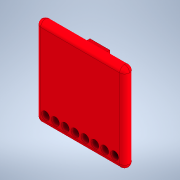
# Autodesk Inventor part: Czujnik GPS ZOE-M8Q
Saved by Autodesk Inventor 2020 (Build 240168000, 168)
## iProperties
Created: 2021-10-10
Part Number: Czujnik GPS ZOE-M8Q
Material: Ogólny
Document SubType Name: Modeling
Designer: Komputer
Density: 1 g/cm^3
Appearance: Domyślna
Author: Komputer
Autodesk Inventor part; units mm, degrees
ref_plane "YZ Plane" through (0, 0, 0) normal (1, 0, 0) x (0, 1, 0)
ref_plane "XZ Plane" through (0, 0, 0) normal (0, 1, 0) x (-1, 0, 0)
ref_plane "XY Plane" through (0, 0, 0) normal (0, 0, 1) x (1, 0, 0)
sketch "Szkic1" plane through (0, 0, 0) normal (0, 0, 1) x (1, 0, 0)
  line L0 (0, 2.25) -> (2.25, 2.25)
  line L1 (2.25, 2.25) -> (2.25, -2.25)
  line L2 (2.25, -2.25) -> (-2.25, -2.25)
  line L3 (-2.25, -2.25) -> (-2.25, 2.25)
  line L4 (-2.25, 2.25) -> (0, 2.25)
  point P0 (0, 0)
  dimension "d2" = 2.25
  dimension "d3" = 4.5
  dimension "d5" = 4.5
  constraints: 10 end point, 3 perpendicular, 2 horizontal
  measures "d2" distance of L0.start L0.end
  measures "d3" distance of L0.end L1.end
  measures "d5" distance of L1.end L2.end
extrude "Wyciągnięcie proste1" add sketch "Szkic1" along normal blind 0.5
fillet "Zaokrąglenie1" radius 0.25 14 edges at (0, -2.25, 0.5) (-2.25, 0, 0.5) (-2.25, 0, 0) (0, -2.25, 0) (-2.25, -2.25, 0.25) (2.25, -2.25, 0.25) (2.25, 0, 0.5) (2.25, 0, 0) (2.25, 2.25, 0.25) (-1.125, 2.25, 0.5) (1.125, 2.25, 0.5) (-1.125, 2.25, 0) (1.125, 2.25, 0) (-2.25, 2.25, 0.25)
sketch "Szkic2" plane through (0, 0, 0) normal (0, 0, -1) x (-1, 0, 0)
  line L0 (-0.75, -0.75) -> (0.75, -0.75)
  line L1 (0.75, -0.75) -> (0.75, 0.75)
  line L2 (0.75, 0.75) -> (-0.75, 0.75)
  line L3 (-0.75, 0.75) -> (-0.75, -0.75)
  line L4 (-0.75, -0.75) -> (0.75, 0.75) construction
  line L5 (0.75, -0.75) -> (-0.75, 0.75) construction
  line L6 (0.5, 1.25) -> (-0.5, 1.25)
  line L7 (-0.5, 1.25) -> (-0.5, 1.75)
  line L8 (-0.5, 1.75) -> (0.5, 1.75)
  line L9 (0.5, 1.75) -> (0.5, 1.25)
  line L10 (0.5, 1.25) -> (-0.5, 1.75) construction
  line L11 (-0.5, 1.25) -> (0.5, 1.75) construction
  point P0 (0, 0)
  point P1 (0, 1.5)
  dimension "d9" = 1.5
  dimension "d10" = 1.5
  dimension "d13" = 1
  dimension "d14" = 0.5
  constraints: 24 end point, 4 midpoint, 4 parallel, 2 horizontal, 2 perpendicular
  measures "d9" distance of L2.end L1.end
  measures "d10" distance of L1.end L0.end
  measures "d13" distance of L7.end L8.end
  measures "d14" distance of L6.end L7.end
extrude "Wyciągnięcie proste2" add sketch "Szkic2" along normal blind 0.25 contours L3 L2 L1 L0
sketch "Szkic3" plane through (0, 0, 0) normal (0, 0, -1) x (-1, 0, 0)
  line L0 (0.5, 1.75) -> (-0.5, 1.75)
  line L1 (-0.5, 1.75) -> (-0.5, 1.25)
  line L2 (-0.5, 1.25) -> (0.5, 1.25)
  line L3 (0.5, 1.25) -> (0.5, 1.75)
  line L4 (0.5, 1.75) -> (-0.5, 1.25) construction
  line L5 (-0.5, 1.75) -> (0.5, 1.25) construction
  point P0 (0, 0)
  point P1 (0, 1.5)
  dimension "d15" = 1
  dimension "d16" = 0.5
  constraints: 12 end point, 2 midpoint, 2 parallel, 1 horizontal, 1 perpendicular
  measures "d15" distance of L2.end L1.end
  measures "d16" distance of L1.end L0.end
extrude "Wyciągnięcie proste3" add sketch "Szkic3" along normal blind 0.5
sketch "Szkic4" plane through (0, 0, 0) normal (0, 0, -1) x (-1, 0, 0)
  line L0 (2, -2) -> (-2, -2) projected
  line L1 (2, -2) -> (2, -1.75)
  line L2 (2, 2) -> (2, -2) projected
  line L3 (2, -1.75) -> (1.75, -1.75)
  circle A0 centre (1.75, -1.75) radius 0.2
  line L4 (1.75, -1.75) -> (1.25, -1.75)
  line L5 (1.25, -1.75) -> (0.75, -1.75)
  line L6 (0.75, -1.75) -> (0.25, -1.75)
  line L7 (0.25, -1.75) -> (-0.25, -1.75)
  line L8 (-0.25, -1.75) -> (-0.75, -1.75)
  line L9 (-0.75, -1.75) -> (-1.25, -1.75)
  line L10 (-1.25, -1.75) -> (-1.75, -1.75)
  circle A1 centre (1.25, -1.75) radius 0.2
  circle A2 centre (0.75, -1.75) radius 0.2
  circle A3 centre (0.25, -1.75) radius 0.2
  circle A4 centre (-0.25, -1.75) radius 0.2
  circle A5 centre (-0.75, -1.75) radius 0.2
  circle A6 centre (-1.25, -1.75) radius 0.2
  circle A7 centre (-1.75, -1.75) radius 0.2
  point P0 (0, 0)
  dimension "d19" = 0.25
  dimension "d20" = 0.25
  dimension "d21" = 0.4
  dimension "d22" = 0.5
  dimension "d23" = 0.5
  dimension "d24" = 0.5
  dimension "d25" = 0.5
  dimension "d26" = 0.5
  dimension "d27" = 0.5
  dimension "d28" = 0.5
  dimension "d29" = 0.4
  dimension "d30" = 0.4
  dimension "d31" = 0.4
  dimension "d32" = 0.4
  dimension "d33" = 0.4
  dimension "d34" = 0.4
  dimension "d35" = 0.4
  constraints: 18 end point, 8 centre point, 8 coincident, 7 point on line, 1 horizontal, 1 perpendicular
  measures "d19" distance of L0.start L1.end
  measures "d20" distance of L1.end L3.end
  measures "d21" diameter of A0
  measures "d22" distance of L4.start L4.end
  measures "d23" distance of L4.end L5.end
  measures "d24" distance of L5.end L6.end
  measures "d25" distance of L6.end L7.end
  measures "d26" distance of L7.end L8.end
  measures "d27" distance of L8.end L9.end
  measures "d28" distance of L9.end L10.end
  measures "d29" diameter of A1
  measures "d30" diameter of A2
  measures "d31" diameter of A3
  measures "d32" diameter of A4
  measures "d33" diameter of A5
  measures "d34" diameter of A6
  measures "d35" diameter of A7
extrude "Wyciągnięcie proste4" cut sketch "Szkic4" against normal blind 0.5
